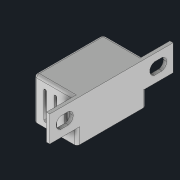
# Autodesk Inventor part: SCDHolder3
Saved by Autodesk Inventor 2021 (Build 250183000, 183)
## iProperties
Created: 2021-05-17
Part Number: SCDHolder3
Material: Generic
Document SubType Name: Modeling
Designer: Adriann Liceralde
Density: 1 g/cm^3
Appearance: Default
Author: Adriann Liceralde
Autodesk Inventor part; units mm, degrees
ref_plane "YZ Plane" through (0, 0, 0) normal (1, 0, 0) x (0, 1, 0)
ref_plane "XZ Plane" through (0, 0, 0) normal (0, 1, 0) x (-1, 0, 0)
ref_plane "XY Plane" through (0, 0, 0) normal (0, 0, 1) x (1, 0, 0)
sketch "Sketch1" plane through (0, 0, 0) normal (0, 0, 1) x (1, 0, 0)
  line L0 (0, 0) -> (95, 0)
  line L1 (95, 0) -> (95, 20)
  line L2 (95, 20) -> (0, 20)
  line L3 (0, 20) -> (0, 0)
  line L4 (8.5, 14.5) -> (14.5, 14.5)
  line L5 (18, 10.2244) -> (18, 9.7756)
  line L6 (14.5, 5.5) -> (8.5, 5.5)
  line L7 (5, 9.7756) -> (5, 10.2244)
  line L8 (11.5, 14.5) -> (8.5, 14.5)
  arc A0 (8.5, 14.5) -> (5, 10) centre (9.4986, 10.1122) ccw
  arc A1 (5, 10) -> (8.5, 5.5) centre (9.4986, 9.8878) ccw
  arc A2 (18, 10) -> (14.5, 14.5) centre (13.5014, 10.1122) ccw
  arc A3 (14.5, 5.5) -> (18, 10) centre (13.5014, 9.8878) ccw
  line L9 (86.5, 14.5) -> (80.5, 14.5)
  line L10 (77, 10.2244) -> (77, 9.7756)
  line L11 (80.5, 5.5) -> (86.5, 5.5)
  line L12 (90, 9.7756) -> (90, 10.2244)
  line L13 (83.5, 14.5) -> (86.5, 14.5)
  arc A4 (90, 10) -> (86.5, 14.5) centre (85.5014, 10.1122) ccw
  arc A5 (86.5, 5.5) -> (90, 10) centre (85.5014, 9.8878) ccw
  arc A6 (80.5, 14.5) -> (77, 10) centre (81.4986, 10.1122) ccw
  arc A7 (77, 10) -> (80.5, 5.5) centre (81.4986, 9.8878) ccw
  point P0 (47.5, 10)
  point P1 (11.5, 10)
  point P2 (83.5, 10)
  dimension "d0" = 95
  dimension "d1" = 20
  constraints: 28 end point, 24 point on circle, 8 centre point, 4 parallel, 2 horizontal, 2 perpendicular
  measures "d0" distance of L2.end L1.end
  measures "d1" distance of L1.end L0.end
extrude "Extrusion1" add sketch "Sketch1" along normal blind 2.5
sketch "Sketch2" plane through (0, 20, 0) normal (0, 1, 0) x (1, 0, 0)
  line L0 (0, 0) -> (95, 0) projected
  line L1 (47.5, 0) -> (21, 0)
  line L2 (47.5, 0) -> (74, 0) construction
  line L3 (47.5, 0) -> (74, 0)
  line L4 (47.5, 0) -> (74, 0) construction
  line L5 (74, 0) -> (74, -2.5)
  line L6 (0, -2.5) -> (95, -2.5) projected
  line L7 (21, 0) -> (21, -2.5)
  line L8 (21, -2.5) -> (74, -2.5)
  constraints: 14 end point, 4 collinear, 2 horizontal, 1 midpoint, 1 parallel, 1 perpendicular, 1 point on line, 1 vertical
extrude "Extrusion2" add sketch "Sketch2" along normal blind 12
sketch "Sketch3" plane through (0, 0, 2.5) normal (0, 0, 1) x (1, 0, 0)
  line L0 (74, 32) -> (21, 32) projected
  line L1 (0, 0) -> (95, 0) projected
  line L2 (21, 32) -> (23.5, 32)
  line L3 (23.5, 32) -> (23.5, 2.5)
  line L4 (23.5, 0) -> (21, 0)
  line L5 (21, 0) -> (21, 32)
  line L6 (74, 20) -> (74, 32) projected
  line L7 (74, 20) -> (74, 0)
  line L8 (74, 0) -> (71.5, 0)
  line L9 (71.5, 2.5) -> (71.5, 32)
  line L10 (71.5, 32) -> (74, 32)
  line L11 (74, 32) -> (74, 0)
  line L12 (23.5, 0) -> (71.5, 0)
  line L13 (71.5, 2.5) -> (23.5, 2.5)
  constraints: 22 end point, 5 parallel, 3 horizontal, 3 perpendicular, 3 point on line
extrude "Extrusion3" add sketch "Sketch3" along normal blind 30.5 contours L6 L7 L1 L5 L0 L3 L13 L9
sketch "Sketch4" plane through (23.5, 2.5, 2.5) normal (0, 1, 0) x (1, 0, 0)
  line L0 (48, -30.5) -> (0, -30.5) projected
  line L1 (48, 0) -> (48, -30.5) projected
  line L2 (0, -30.5) -> (48, -30.5)
  line L3 (48, -30.5) -> (48, -28)
  line L4 (48, -28) -> (0, -28)
  line L5 (0, -28) -> (0, -30.5)
  point P0 (-23.5, 2.5)
  dimension "d24" = 2.5
  constraints: 8 end point, 2 parallel, 1 horizontal, 1 perpendicular, 1 point on line
  measures "d24" distance of L3.end L2.end
extrude "Extrusion4" add sketch "Sketch4" along normal up to surface (29.5 mm away)
sketch "Sketch5" plane through (23.5, 2.5, 2.5) normal (1, 0, 0) x (0, 0, -1)
  line L0 (0, 0) -> (-28, 0) projected
  line L1 (-14, 0) -> (-14, 29.5)
  line L2 (0, 29.5) -> (-28, 29.5) projected
  line L3 (-15, 14.75) -> (-15, 24.75)
  line L4 (-15, 14.75) -> (-15, 4.75)
  line L5 (-13, 14.75) -> (-13, 4.75)
  line L6 (-13, 14.75) -> (-13, 24.75)
  arc A0 (-13, 24.75) -> (-15, 24.75) centre (-14, 24.75) ccw
  arc A1 (-15, 4.75) -> (-13, 4.75) centre (-14, 4.75) ccw
  line L7 (-14, 14.75) -> (-14, 15.75)
  line L8 (-15, 14.75) -> (-13, 14.75)
  line L9 (-23, 14.75) -> (-23, 24.75)
  line L10 (-21, 14.75) -> (-21, 24.75)
  line L11 (-21, 14.75) -> (-21, 4.75)
  line L12 (-23, 14.75) -> (-23, 4.75)
  arc A2 (-23, 4.75) -> (-21, 4.75) centre (-22, 4.75) ccw
  arc A3 (-21, 24.75) -> (-23, 24.75) centre (-22, 24.75) ccw
  line L13 (-6, 14.75) -> (-6, 15.75)
  line L14 (-7, 14.75) -> (-7, 4.75)
  line L15 (-5, 14.75) -> (-5, 4.75)
  arc A4 (-7, 4.75) -> (-5, 4.75) centre (-6, 4.75) ccw
  line L16 (-7, 14.75) -> (-7, 24.75)
  line L17 (-5, 14.75) -> (-5, 24.75)
  arc A5 (-5, 24.75) -> (-7, 24.75) centre (-6, 24.75) ccw
  point P0 (2.5, -2.5)
  dimension "d38" = 8
  dimension "d45" = 8
  constraints: 32 end point, 12 point on circle, 6 centre point, 4 tangent, 3 horizontal, 3 midpoint, 3 vertical, 1 perpendicular, 1 point on line, 31 other
  measures "d38" distance of L3.start L9.start
  measures "d45" distance of L7.end L13.end
extrude "Extrusion5" cut sketch "Sketch5" along normal through all both and the other way through all
sketch "Sketch8" plane through (71.5, 2.5, 30.5) normal (0, 0, -1) x (-1, 0, 0)
  line L0 (-2.5, 29.5) -> (50.5, 29.5) projected
  line L1 (48, 0) -> (0, 0) projected
  line L2 (24, 29.5) -> (53.5, 29.5) construction
  line L3 (23.9997, 15.0133) -> (24.9997, 15.0133) construction
  line L4 (22.9997, 15.0133) -> (22.9997, 25.0133)
  line L5 (22.9997, 15.0133) -> (22.9997, 5.0133)
  line L6 (24.9997, 15.0133) -> (24.9997, 5.0133)
  line L7 (24.9997, 15.0133) -> (24.9997, 25.0133)
  arc A0 (24.9997, 25.0133) -> (22.9997, 25.0133) centre (23.9997, 25.0393) ccw
  arc A1 (22.9997, 5.0133) -> (24.9997, 5.0133) centre (23.9997, 4.9873) ccw
  line L8 (30.9997, 15.0133) -> (30.9997, 25.0133)
  line L9 (30.9997, 15.0133) -> (30.9997, 5.0133)
  line L10 (32.9997, 15.0133) -> (32.9997, 5.0133)
  line L11 (32.9997, 15.0133) -> (32.9997, 25.0133)
  arc A2 (32.9997, 25.0133) -> (30.9997, 25.0133) centre (31.9997, 25.0393) ccw
  arc A3 (30.9997, 5.0133) -> (32.9997, 5.0133) centre (31.9997, 4.9873) ccw
  line L12 (38.9997, 15.0133) -> (38.9997, 25.0133)
  line L13 (38.9997, 15.0133) -> (38.9997, 5.0133)
  line L14 (40.9997, 15.0133) -> (40.9997, 5.0133)
  line L15 (40.9997, 15.0133) -> (40.9997, 25.0133)
  arc A4 (40.9997, 25.0133) -> (38.9997, 25.0133) centre (39.9997, 25.0393) ccw
  arc A5 (38.9997, 5.0133) -> (40.9997, 5.0133) centre (39.9997, 4.9873) ccw
  line L16 (14.9997, 15.0133) -> (14.9997, 25.0133)
  line L17 (16.9997, 15.0133) -> (16.9997, 25.0133)
  arc A6 (16.9997, 25.0133) -> (14.9997, 25.0133) centre (15.9997, 25.0393) ccw
  line L18 (14.9997, 15.0133) -> (14.9997, 5.0133)
  line L19 (16.9997, 15.0133) -> (16.9997, 5.0133)
  arc A7 (14.9997, 5.0133) -> (16.9997, 5.0133) centre (15.9997, 4.9873) ccw
  line L20 (6.9997, 15.0133) -> (6.9997, 25.0133)
  line L21 (8.9997, 15.0133) -> (8.9997, 25.0133)
  arc A8 (8.9997, 25.0133) -> (6.9997, 25.0133) centre (7.9997, 25.0393) ccw
  line L22 (6.9997, 15.0133) -> (6.9997, 5.0133)
  line L23 (8.9997, 15.0133) -> (8.9997, 5.0133)
  arc A9 (6.9997, 5.0133) -> (8.9997, 5.0133) centre (7.9997, 4.9873) ccw
  point P0 (71.5, -2.5)
  point P1 (31.9997, 15.0133)
  point P2 (39.9997, 15.0133)
  point P3 (15.9997, 15.0133)
  point P4 (22.9997, 25.0133)
  point P5 (24.9997, 25.0133)
  point P6 (7.9997, 15.0133)
  point P7 (14.9997, 25.0133)
  point P8 (15.9997, 25.0393)
  dimension "d64" = 8
  dimension "d71" = 8
  constraints: 44 end point, 20 point on circle, 10 centre point, 4 horizontal, 4 vertical, 1 midpoint, 66 other
  measures "d64" distance of L3.start point (32, 15.013)
  measures "d71" distance of L3.start point (16, 15.013)
extrude "Extrusion6" cut sketch "Sketch8" against normal up to surface (2.5 mm away)
fillet "Fillet1" radius 2 4 edges at (74, 16, 33) (21, 16, 33) (74, 26, 0) (21, 26, 0)
fillet "Fillet2" radius 2 5 edges at (73.4142, 0, 32.4142) (74, 0, 16.75) (21.5858, 0, 32.4142) (21, 0, 16.75) (47.5, 0, 33)
body "Solid1"
